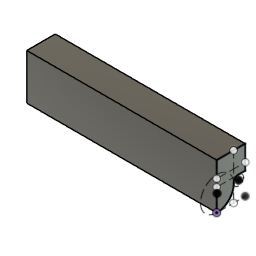
HTD-3M Belt (Autodesk Fusion 360 design; units mm, degrees)
Autodesk Fusion 360 part; units mm, degrees
sketch "Sketch1" plane through (0, 0, 0) normal (1, 0, 0) x (0, 1, 0)
  line L0 (0, 0) -> (0, 2.4) construction
  line L1 (0, 0) -> (1.5, 0) construction
  line L2 (0, 1.17) -> (1.5, 1.17)
  line L3 (0, 1.551) -> (1.5, 1.551) construction
  line L4 (0.89, 0) -> (0.89, 2.4) construction
  line L5 (0, 2.4) -> (1.5, 2.4) construction
  circle A0 centre (1.15, 0.91) radius 0.26 construction
  circle A1 centre (0.02, 0.87) radius 0.87 construction
  line L6 (0, 2.4) -> (0, 0)
  line L7 (1.5, 1.17) -> (1.5, 2.4)
  line L8 (0, 2.4) -> (1.5, 2.4)
  line L9 (1.5, 1.17) -> (1.15, 1.17)
  arc A2 (0, 0) -> (0.89, 0.91) centre (0.0204, 0.8702) ccw
  arc A3 (1.15, 1.17) -> (0.89, 0.91) centre (1.15, 0.91) ccw
  dimension "d1" = 2.4
  dimension "d3" = 1.5
  dimension "d4" = -1.17
  dimension "d5" = -1.551
  dimension "d6" = 0.89
  dimension "d8" = 0.381
  dimension "d9" = 1.5
  dimension "d10" = 0.52
  dimension "d11" = 0.87
  constraint coincident L0.start L1.start
  constraint vertical L0
  constraint perpendicular L0 L1
  constraint perpendicular L0 L5
  constraint tangent L2 A0
  constraint tangent L4 A0
  constraint tangent L4 A1
  constraint tangent L1 A1
  constraint perpendicular L2 L7
  constraint coincident A0 L9.end
  constraint tangent A0 L9
  constraint tangent A1 A2
  constraint coincident A0 A2.end
  constraint coincident L4 A2.end
  constraint tangent L9 A3
  measures "d1" distance of L0.start L0.end
  measures "d3" distance of L0.start L1.end
  measures "d8" distance of L2 L3
  measures "d9" distance of L0.end L5.end
  measures "d10" diameter of A0
  measures "d11" radius of A1
extrude "Extrude1" add sketch "Sketch1" against normal blind 10
equation "d5 = -1.17 mm - 0.381 mm"
equation "d6 = ( 1.78 / 2 ) * 1 mm"
equation "d10 = ( 0.26 * 2 ) * 1 mm"
